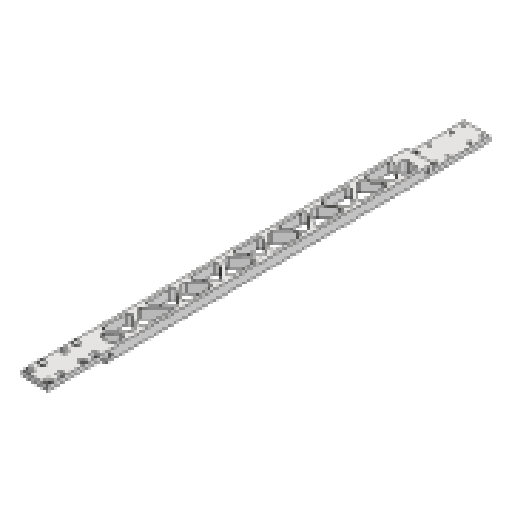
# Autodesk Inventor part: mgn7 300mm Connector Plate
Saved by Autodesk Inventor 2023 (Build 270158000, 158)
## iProperties
Created: 2022-09-25
Part Number: mgn7 300mm Connector Plate
Material: Generic
Document SubType Name: Modeling
Designer: deli
Density: 1 g/cm^3
Appearance: Default
Mass: 15.4529 g
Surface Area: 147.421 cm^2
Volume: 15.4529 cm^3
Author: deli
Autodesk Inventor part; units mm, degrees
ref_plane "YZ Plane" through (0, 0, 0) normal (1, 0, 0) x (0, 1, 0)
ref_plane "XZ Plane" through (0, 0, 0) normal (0, 1, 0) x (-1, 0, 0)
ref_plane "XY Plane" through (0, 0, 0) normal (0, 0, 1) x (1, 0, 0)
sketch "Sketch1" plane through (0, 0, 0) normal (0, 1, 0) x (-1, 0, 0)
  line L0 (25.6456, 340.4178) -> (8.6456, 340.4178)
  line L1 (8.6456, 340.4178) -> (8.6456, 30.4178)
  line L2 (8.6456, 30.4178) -> (25.6456, 30.4178)
  line L3 (25.6456, 30.4178) -> (25.6456, 340.4178)
  circle A0 centre (23.1456, 328.1678) radius 1.1
  circle A1 centre (23.1456, 320.1678) radius 1.1
  circle A2 centre (11.1456, 328.1678) radius 1.1
  circle A3 centre (11.1456, 320.1678) radius 1.1
  line L4 (23.1456, 328.1678) -> (23.1456, 320.1678) construction
  line L5 (23.1456, 320.1678) -> (11.1456, 320.1678) construction
  line L6 (11.1456, 320.1678) -> (11.1456, 328.1678) construction
  line L7 (11.1456, 328.1678) -> (23.1456, 328.1678) construction
  circle A4 centre (23.1456, 305.6678) radius 1.1
  circle A5 centre (23.1456, 297.6678) radius 1.1
  circle A6 centre (11.1456, 305.6678) radius 1.1
  circle A7 centre (11.1456, 297.6678) radius 1.1
  line L8 (23.1456, 305.6678) -> (23.1456, 297.6678) construction
  line L9 (23.1456, 297.6678) -> (11.1456, 297.6678) construction
  line L10 (11.1456, 297.6678) -> (11.1456, 305.6678) construction
  line L11 (11.1456, 305.6678) -> (23.1456, 305.6678) construction
  circle A8 centre (23.1456, 73.1678) radius 1.1
  circle A9 centre (23.1456, 65.1678) radius 1.1
  circle A10 centre (11.1456, 73.1678) radius 1.1
  circle A11 centre (11.1456, 65.1678) radius 1.1
  line L12 (23.1456, 73.1678) -> (23.1456, 65.1678) construction
  line L13 (23.1456, 65.1678) -> (11.1456, 65.1678) construction
  line L14 (11.1456, 65.1678) -> (11.1456, 73.1678) construction
  line L15 (11.1456, 73.1678) -> (23.1456, 73.1678) construction
  circle A12 centre (23.1456, 50.6678) radius 1.1
  circle A13 centre (23.1456, 42.6678) radius 1.1
  circle A14 centre (11.1456, 50.6678) radius 1.1
  circle A15 centre (11.1456, 42.6678) radius 1.1
  line L16 (23.1456, 50.6678) -> (23.1456, 42.6678) construction
  line L17 (23.1456, 42.6678) -> (11.1456, 42.6678) construction
  line L18 (11.1456, 42.6678) -> (11.1456, 50.6678) construction
  line L19 (11.1456, 50.6678) -> (23.1456, 50.6678) construction
  point P0 (0, 0)
  point P1 (17.1456, 30.4178)
  dimension "d0" = 17
  dimension "d23" = 2.2
  dimension "d24" = 2.2
  dimension "d25" = 2.2
  dimension "d26" = 2.2
  dimension "d27" = 12
  dimension "d28" = 8
  dimension "d29" = 2.5
  dimension "d31" = 2.2
  dimension "d32" = 2.2
  dimension "d33" = 2.2
  dimension "d34" = 2.2
  dimension "d35" = 8
  dimension "d36" = 12
  dimension "d38" = 14.5
  dimension "d49" = 8
  dimension "d50" = 12
  dimension "d58" = 8
  dimension "d59" = 12
  dimension "d63" = 14.5
  dimension "d94" = 224.5
  dimension "d101" = 285.5
  dimension "d107" = 12.25
  dimension "d108" = 12.25
  dimension "d213" = 2.5
  dimension "d214" = 2.5
  dimension "d215" = 2.5
  constraints: 40 end point, 16 centre point, 12 perpendicular, 8 equal radius, 4 vertical, 3 horizontal, 3 parallel, 1 midpoint
  measures "d0" distance of L2.end L1.end
  measures "d23" diameter of A0
  measures "d24" diameter of A1
  measures "d25" diameter of A2
  measures "d26" diameter of A3
  measures "d27" distance of L6.end L4.start
  measures "d28" distance of L4.start L4.end
  measures "d29" distance from line of L1 L6.end
  measures "d31" diameter of A4
  measures "d32" diameter of A5
  measures "d33" diameter of A6
  measures "d34" diameter of A7
  measures "d35" distance of L8.start L8.end
  measures "d36" distance of L10.end L8.start
  measures "d38" distance of L10.end L5.end
  measures "d49" distance of L12.end L15.end
  measures "d50" distance of L15.start L15.end
  measures "d58" distance of L19.end L16.end
  measures "d59" distance of L19.start L19.end
  measures "d63" distance of L14.start L19.start
  measures "d94" distance between parallel lines of L15 L9
  measures "d101" distance of L18.start L6.end
  measures "d107" distance from line of point (17.146, 30.418) L17
  measures "d108" distance between parallel lines of L0 L7
  measures "d213" distance between parallel lines of L1 L18
  measures "d214" distance between parallel lines of L1 L14
  measures "d215" distance between parallel lines of L1 L10
extrude "Extrusion1" add sketch "Sketch1" along normal blind 6.35
sketch "Sketch2" plane through (0, 6.35, 0) normal (0, 1, 0) x (1, 0, 0)
  line L0 (-8.6456, -340.4178) -> (-8.6456, -30.4178) projected
  line L1 (-25.6456, -30.4178) -> (-25.6456, -340.4178) projected
  line L2 (-8.6456, -35.4178) -> (-25.6456, -35.4178)
  line L3 (-25.6456, -35.4178) -> (-25.6456, -80.4178)
  line L4 (-25.6456, -80.4178) -> (-8.6456, -80.4178)
  line L5 (-8.6456, -80.4178) -> (-8.6456, -35.4178)
  line L6 (-8.6456, -30.4178) -> (-25.6456, -30.4178) projected
  point P0 (0, 0)
  point P1 (-8.6456, -80.4178)
  point P2 (-25.6456, -35.4178)
  dimension "d278" = 45
  dimension "d279" = 5
  constraints: 8 end point, 2 parallel, 2 point on line, 1 horizontal, 1 perpendicular
  measures "d278" distance between parallel lines of L4 L2
  measures "d279" distance between parallel lines of L6 L2
extrude "Extrusion2" cut sketch "Sketch2" against normal blind 2.2 contours L4 L1 L2 L0
sketch "Sketch3" plane through (0, 0, 0) normal (0, -1, 0) x (1, 0, 0)
  line L0 (-8.6456, 290.4178) -> (-25.6456, 290.4178)
  line L1 (-25.6456, 290.4178) -> (-25.6456, 335.4178)
  line L2 (-25.6456, 335.4178) -> (-8.6456, 335.4178)
  line L3 (-8.6456, 335.4178) -> (-8.6456, 290.4178)
  line L4 (-8.6456, 340.4178) -> (-8.6456, 30.4178) projected
  line L5 (-25.6456, 340.4178) -> (-8.6456, 340.4178) projected
  point P0 (0, 0)
  dimension "d280" = 45
  dimension "d281" = 5
  constraints: 8 end point, 2 parallel, 1 collinear, 1 horizontal, 1 perpendicular
  measures "d280" distance between parallel lines of L2 L0
  measures "d281" distance between parallel lines of L5 L2
extrude "Extrusion3" cut sketch "Sketch3" against normal blind 2.2
sketch "Sketch5" plane through (0, 6.35, 0) normal (0, 1, 0) x (1, 0, 0)
  line L0 (-8.6456, -70.9178) -> (-25.6456, -70.9178) projected
  line L1 (-8.6456, -302.6178) -> (-25.6456, -302.6178) projected
  line L2 (-25.6456, -302.6178) -> (-25.6456, -70.9178)
  line L3 (-8.6456, -70.9178) -> (-8.6456, -302.6178)
  line L4 (-23.6456, -95.8817) -> (-23.6456, -119.2922)
  line L5 (-23.6456, -119.2922) -> (-10.6456, -107.5869)
  line L6 (-10.6456, -107.5869) -> (-23.6456, -95.8817)
  line L7 (-23.6456, -93.1904) -> (-10.6456, -93.1904)
  line L8 (-10.6456, -93.1904) -> (-10.6456, -104.8956)
  line L9 (-10.6456, -104.8956) -> (-23.6456, -93.1904)
  line L10 (-10.6456, -110.2782) -> (-23.6456, -121.9834)
  line L11 (-23.6456, -121.9834) -> (-10.6456, -133.6887)
  line L12 (-10.6456, -133.6887) -> (-10.6456, -110.2782)
  line L13 (-23.6456, -124.6747) -> (-10.6456, -136.3799)
  line L14 (-10.6456, -136.3799) -> (-23.6456, -148.0852)
  line L15 (-23.6456, -148.0852) -> (-23.6456, -124.6747)
  line L16 (-10.6456, -139.0712) -> (-23.6456, -150.7765)
  line L17 (-23.6456, -150.7765) -> (-10.6456, -162.4817)
  line L18 (-10.6456, -162.4817) -> (-10.6456, -139.0712)
  line L19 (-23.6456, -153.4677) -> (-10.6456, -165.173)
  line L20 (-10.6456, -165.173) -> (-23.6456, -176.8782)
  line L21 (-23.6456, -176.8782) -> (-23.6456, -153.4677)
  line L22 (-10.6456, -167.8643) -> (-23.6456, -179.5695)
  line L23 (-23.6456, -179.5695) -> (-10.6456, -191.2748)
  line L24 (-10.6456, -191.2748) -> (-10.6456, -167.8643)
  line L25 (-23.6456, -182.2608) -> (-23.6456, -205.6713)
  line L26 (-23.6456, -205.6713) -> (-10.6456, -193.966)
  line L27 (-10.6456, -193.966) -> (-23.6456, -182.2608)
  line L28 (-10.6456, -196.6573) -> (-23.6456, -208.3625)
  line L29 (-23.6456, -208.3625) -> (-10.6456, -220.0678)
  line L30 (-10.6456, -220.0678) -> (-10.6456, -196.6573)
  line L31 (-23.6456, -211.0538) -> (-10.6456, -222.7591)
  line L32 (-10.6456, -222.7591) -> (-23.6456, -234.4643)
  line L33 (-23.6456, -234.4643) -> (-23.6456, -211.0538)
  line L34 (-7.6456, -67.1678) -> (-7.6456, -282.1678)
  line L35 (-10.6456, -225.4503) -> (-23.6456, -237.1556)
  line L36 (-23.6456, -237.1556) -> (-10.6456, -248.8608)
  line L37 (-10.6456, -248.8608) -> (-10.6456, -225.4503)
  line L38 (-23.6456, -239.8468) -> (-10.6456, -251.5521)
  line L39 (-10.6456, -251.5521) -> (-23.6456, -263.2573)
  line L40 (-23.6456, -263.2573) -> (-23.6456, -239.8468)
  line L41 (-6.6456, -66.1678) -> (-6.6456, -281.1678)
  line L42 (-10.6456, -254.2434) -> (-23.6456, -265.9486)
  line L43 (-23.6456, -265.9486) -> (-10.6456, -277.6539)
  line L44 (-10.6456, -277.6539) -> (-10.6456, -254.2434)
  line L45 (-23.6456, -268.6399) -> (-10.6456, -280.3451)
  line L46 (-23.6456, -280.3451) -> (-23.6456, -268.6399)
  line L47 (-10.6456, -280.3451) -> (-23.6456, -280.3451)
  point P0 (0, 0)
  point P1 (-10.6456, -188.3577)
  point P2 (-10.6456, -154.3183)
  point P3 (-23.6456, -306.5944)
  dimension "d216" = 48
  dimension "d217" = 2
  dimension "d218" = 2
  dimension "d219" = 22.2726
  dimension "d221" = 2
  dimension "d227" = 2
  dimension "d228" = 2
  dimension "d232" = 2
  dimension "d233" = 2
  dimension "d234" = 231.7
  dimension "d235" = 2
  dimension "d236" = 2
  dimension "d237" = 2
  dimension "d238" = 2
  dimension "d244" = 2
  dimension "d252" = 2
  dimension "d253" = 2
  dimension "d262" = 2
  dimension "d266" = 187.1547
  constraints: 92 end point, 27 parallel, 21 point on line, 13 equal length, 5 collinear, 3 perpendicular, 2 vertical, 1 horizontal
  measures "d216" angle of L6 L4
  measures "d217" distance between parallel lines of L2 L4
  measures "d218" distance between parallel lines of L3 L8
  measures "d219" distance between parallel lines of L0 L7
  measures "d221" distance from line of L6 L7.start
  measures "d227" distance between parallel lines of L10 L5
  measures "d228" distance between parallel lines of L11 L13
  measures "d232" distance between parallel lines of L16 L14
  measures "d233" distance between parallel lines of L17 L19
  measures "d234" distance between parallel lines of L1 L0
  measures "d235" distance between parallel lines of L22 L20
  measures "d236" distance between parallel lines of L23 L27
  measures "d237" distance between parallel lines of L28 L26
  measures "d238" distance between parallel lines of L29 L31
  measures "d244" distance between parallel lines of L36 L38
  measures "d252" distance between parallel lines of L35 L32
  measures "d253" distance between parallel lines of L43 L45
  measures "d262" distance between parallel lines of L39 L42
  measures "d266" distance between parallel lines of L47 L7
extrude "Extrusion5" cut sketch "Sketch5" against normal blind 10 contours L6 L5 L4 | L7 L8 L9 | L12 L11 L10 | L13 L14 L15 | L18 L17 L16 | L19 L20 L21 | L24 L23 L22 | L27 L26 L25 | L30 L29 L28 | L31 L32 L33 | L37 L36 L35 | L38 L39 L40 | L44 L43 L42 | L45 L47 L46
fillet "Fillet3" radius 2 41 edges at (-23.6456, 3.175, 234.4643) (-10.6456, 3.175, 222.7591) (-23.6456, 3.175, 211.0538) (-23.6456, 3.175, 208.3625) (-10.6456, 3.175, 220.0678) (-10.6456, 3.175, 196.6573) (-23.6456, 3.175, 205.6713) (-10.6456, 3.175, 193.966) (-23.6456, 3.175, 182.2608) (-23.6456, 3.175, 179.5695) (-10.6456, 3.175, 191.2748) (-10.6456, 3.175, 167.8643) (-23.6456, 3.175, 176.8782) (-10.6456, 3.175, 165.173) (-23.6456, 3.175, 153.4677) (-23.6456, 3.175, 150.7765) (-23.6456, 3.175, 148.0852) (-10.6456, 3.175, 162.4817) (-10.6456, 3.175, 139.0712) (-10.6456, 3.175, 136.3799) (-10.6456, 3.175, 133.6887) (-23.6456, 3.175, 124.6747) (-23.6456, 3.175, 121.9834) (-23.6456, 3.175, 119.2922) (-10.6456, 3.175, 110.2782) (-10.6456, 3.175, 107.5869) (-10.6456, 3.175, 104.8956) (-23.6456, 3.175, 95.8817) (-23.6456, 3.175, 93.1904) (-10.6456, 3.175, 93.1904) (-10.6456, 3.175, 225.4503) (-23.6456, 3.175, 237.1556) (-10.6456, 3.175, 248.8608) (-10.6456, 3.175, 251.5521) (-23.6456, 3.175, 239.8468) (-23.6456, 3.175, 265.9486) (-23.6456, 3.175, 263.2573) (-23.6456, 3.175, 268.6399) (-10.6456, 3.175, 277.6539) (-10.6456, 3.175, 280.3451) (-23.6456, 3.175, 280.3451)
chamfer "Chamfer1" distance 1.2 angle 45 16 edges at (-10.0456, 6.35, 328.1678) (-22.0456, 6.35, 328.1678) (-22.0456, 6.35, 320.1678) (-10.0456, 6.35, 320.1678) (-22.0456, 6.35, 305.6678) (-10.0456, 6.35, 305.6678) (-22.0456, 6.35, 297.6678) (-10.0456, 6.35, 297.6678) (-22.0456, 0, 73.1678) (-10.0456, 0, 65.1678) (-10.0456, 0, 73.1678) (-10.0456, 0, 50.6678) (-10.0456, 0, 42.6678) (-22.0456, 0, 42.6678) (-22.0456, 0, 50.6678) (-22.0456, 0, 65.1678)
sketch "Sketch6" plane through (-25.6456, 6.35, 70.9178) normal (-1, 0, 0) x (0, 0, 1)
  circle A0 centre (-38, -3.85) radius 1.5
  line L0 (-40.5, 0) -> (269.5, 0) projected
  circle A1 centre (267, -2.5) radius 1.5
  line L1 (-40.5, -6.35) -> (-40.5, 0) projected
  line L2 (269.5, -6.35) -> (269.5, 0) projected
  line L3 (-40.5, -6.35) -> (219.5, -6.35) projected
  point P0 (-70.9178, -6.35)
  dimension "d267" = 3
  dimension "d282" = 2.5
  dimension "d283" = 2.5
  dimension "d284" = 1
  dimension "d285" = 1
  constraints: 2 centre point, 1 equal radius
  measures "d267" diameter of A0
  measures "d282" distance from line of L1 A0.centre
  measures "d283" distance from line of L2 A1.centre
  measures "d284" distance edge to line of A0 L3
  measures "d285" distance edge to line of A1 L0
extrude "Extrusion6" cut sketch "Sketch6" against normal blind 10
thread "Thread4" size "M3x0.5" class "6H" standard "ANSI Metric M Profile" full length
thread "Thread5" size "M3x0.5" class "6H" standard "ANSI Metric M Profile" full length
equation "\"d24\" = d23"
equation "\"d25\" = d23"
equation "\"d26\" = d23"
equation "\"d29\" = -0.5 * d27 + 0.5 * d0"
equation "\"d31\" = d23"
equation "\"d32\" = d23"
equation "\"d33\" = d23"
equation "\"d34\" = d23"
equation "\"d35\" = d28"
equation "\"d36\" = d27"
equation "\"d63\" = d38"
body "Solid1"
